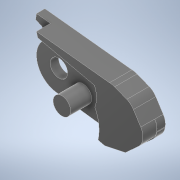
# Autodesk Inventor part: Pieza3
Saved by Autodesk Inventor 2022 (Build 260153000, 153)
## iProperties
Created: 2022-11-04
Part Number: Pieza3
Material: Resina acetálica, negra
Document SubType Name: Modeling
Designer: Mauricio Guerrero
Density: 1.425 g/cm^3
Appearance: Suave - Negro
Author: Mauricio Guerrero
## iProperties of the stored document Pieza3_3DPrint.ipt
Created: 2022-11-06
Part Number: Pieza3_3DPrint
Material: Genérico
Document SubType Name: Modeling
Designer: Mauricio Guerrero
Density: 1 g/cm^3
Appearance: Valor por defecto
Author: Mauricio Guerrero
Autodesk Inventor part; units mm, degrees
ref_plane "YZ Plane" through (0, 0, 0) normal (1, 0, 0) x (0, 1, 0)
ref_plane "XZ Plane" through (0, 0, 0) normal (0, 1, 0) x (-1, 0, 0)
ref_plane "XY Plane" through (0, 0, 0) normal (0, 0, 1) x (1, 0, 0)
sketch "Boceto1" plane through (0, 0, 0) normal (0, 0, 1) x (1, 0, 0)
  circle A0 centre (0, 0) radius 1.25
  arc A1 (-1.6574, 2.7373) -> (-0.4126, -3.1733) centre (0, 0) ccw
  line L0 (7.1, -4.15) -> (7.1, -7.1226) construction
  line L1 (-3.2, 3.2) -> (-3.2, -3.4) construction
  line L2 (-0.4126, -3.1733) -> (7.1, -4.15)
  line L3 (-1.4, 3.8) -> (-1.4, 6.2978) construction
  line L4 (14.1, 2.7373) -> (14.1, -1.982) construction
  line L5 (7.1, -4.15) -> (8.5447, -4.3189)
  line L6 (8.5447, -4.3189) -> (11.6298, -3.6616)
  line L7 (11.6298, -3.6616) -> (13.3209, -2.1424)
  line L8 (13.9587, -0.9739) -> (13.978, -0.8543)
  line L9 (9.9548, 3.6595) -> (11.6833, 2.9749)
  line L10 (12.6312, 2.1939) -> (13.688, 0.5435)
  arc A2 (12.6312, 2.1939) -> (11.6833, 2.9749) centre (10.9469, 1.1154) ccw
  arc A3 (9.9548, 3.6595) -> (9.2184, 3.8) centre (9.2184, 1.8) ccw
  arc A4 (13.978, -0.8543) -> (13.688, 0.5435) centre (12.0037, -0.535) ccw
  arc A5 (13.3209, -2.1424) -> (13.9587, -0.9739) centre (11.9843, -0.6546) ccw
  line L11 (-1.6574, 2.7373) -> (-2.4537, 3.981)
  line L12 (-2.4537, 3.981) -> (-3.3251, 4.3261)
  line L13 (-3.3251, 4.3261) -> (-3.2, 5.1465)
  line L14 (-3.2, 5.1465) -> (9.2184, 3.8)
  point P0 (9.6, 3.8)
  point P1 (14.1, -0.1)
  dimension "d0" = 2.5
  dimension "d4" = 6.4
  dimension "d5" = 4.15
  dimension "d6" = 10.3
  dimension "d7" = 3.8
  dimension "d8" = 1.8
  dimension "d9" = 11
  dimension "d10" = 7
  dimension "d19" = 2
  constraints: 30 end point, 10 point on circle, 9 tangent, 6 centre point, 5 point on line, 4 vertical, 3 equal radius, 2 coincident
  measures "d0" diameter of A0
  measures "d4" diameter of A1
  measures "d5" vertical distance of L0.start point (0, 0)
  measures "d6" distance between parallel lines of L0 L1
  measures "d7" vertical distance of point (0, 0) L3.start
  measures "d8" distance between parallel lines of L1 L3
  measures "d9" distance of L3.start point (9.6, 3.8)
  measures "d10" distance from line of L4 L0.start
  measures "d19" radius of A2
extrude "Extrusión1" add sketch "Boceto1" along normal blind 1.2
sketch "Boceto5" plane through (0, 0, 1.2) normal (0, 0, 1) x (1, 0, 0)
  line L0 (7.5987, -4.0877) -> (8.5447, -4.3189)
  line L1 (8.5447, -4.3189) -> (11.6298, -3.6616)
  line L2 (11.4934, -3.6907) -> (13.3446, -2.0049)
  line L3 (9.9548, 3.6595) -> (11.6833, 2.9749)
  line L4 (12.6312, 2.1939) -> (13.6823, 0.5523)
  arc A0 (12.6312, 2.1939) -> (11.6833, 2.9749) centre (10.9469, 1.1154) ccw
  arc A1 (9.9548, 3.6595) -> (9.2184, 3.8) centre (9.2184, 1.8) ccw
  arc A2 (13.3446, -2.0049) -> (13.6823, 0.5523) centre (11.998, -0.5262) ccw
  arc A3 (3.8787, -10.625) -> (3.8888, -10.616) centre (2.5421, -9.1373) ccw
  arc A4 (7.5987, -4.0877) -> (7.1292, -0.2455) centre (2.0351, -2.8178) ccw
  arc A5 (7.1292, -0.2455) -> (7.0735, 2.4165) centre (3.9271, 1.0191) ccw
  arc A6 (9.9548, 3.6595) -> (9.2184, 3.8) centre (9.2184, 1.8) ccw projected
  line L5 (9.2184, 3.8) -> (5.136, 4.2426)
  line L6 (5.136, 4.2426) -> (-1.2086, 4.9306)
  line L7 (9.2184, 3.8) -> (-3.2, 5.1465) projected
  line L8 (-1.0169, 4.2426) -> (-1.2086, 4.9306)
  line L9 (-1.0169, 4.2426) -> (7.0735, 2.4165)
  point P0 (0, 0)
  point P1 (9.6, 3.8)
  constraints: 18 end point, 12 point on circle, 6 centre point, 6 tangent, 3 equal radius, 3 point on line
extrude "Extrusión5" add sketch "Boceto5" along normal blind 2
sketch "Boceto6" plane through (0, 0, 1.2) normal (0, 0, 1) x (1, 0, 0)
  circle A0 centre (3.427, -1.4569) radius 1.25
  point P0 (0, 0)
  dimension "d26" = 2.5
  constraints: 1 centre point
  measures "d26" diameter of A0
extrude "Extrusión6" add sketch "Boceto6" along normal blind 3
